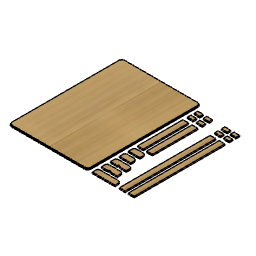
poglos_main_board 211121 (Autodesk Fusion 360 design; units mm, degrees)
Autodesk Fusion 360 part; units mm, degrees
sketch "Main Board" plane through (0, 0, 0) normal (0, 0, 1) x (1, 0, 0)
  line L0 (0, 0) -> (350, 0)
  line L1 (350, 0) -> (350, 500)
  line L2 (350, 500) -> (0, 500)
  line L3 (0, 500) -> (0, 0)
  line L4 (134.9528, 99.915) -> (214.9528, 99.915)
  line L5 (214.9528, 99.915) -> (214.9528, 59.915)
  line L6 (214.9528, 59.915) -> (134.9528, 59.915)
  line L7 (134.9528, 59.915) -> (134.9528, 99.915)
  line L8 (75, 450) -> (275, 450)
  line L9 (275, 450) -> (275, 50)
  line L10 (275, 50) -> (75, 50)
  line L11 (75, 50) -> (75, 450)
  dimension "d1" = 350
  dimension "d2" = 500
  constraint horizontal L0
  constraint vertical L1
  constraint horizontal L2
  constraint vertical L3
  constraint coincident L0.start L3.end
  constraint perpendicular L3 L4
  constraint perpendicular L4 L5
  constraint perpendicular L3 L6
  constraint perpendicular L4 L7
  constraint horizontal L8
  constraint vertical L9
  constraint horizontal L10
  constraint vertical L11
  measures "d1" distance of L0.start L0.end
  measures "d2" distance of L0.start L2.end
extrude "Extrude1" add sketch "Main Board" along normal blind 3 contours L0 L1 L2 L3 | L4 L5 L6 L7 | L8 L9 L10 L11 makes body 1
fillet "Fillet1" radius 15 4 edges at (350, 500, 1.5) (350, 0, 1.5) (0, 0, 1.5) (0, 500, 1.5) on bodies 1
extrude "Extrude2" add 1 faces at (116.6667, 328.3333, 3) along direction (0, 0, 1) blind 3 on bodies 1 bodies 1
chamfer "Chamfer2" distance 2 angle 45 8 edges at (175, 0, 6) (345.6066, 4.3934, 6) (350, 250, 6) (345.6066, 495.6066, 6) (175, 500, 6) (4.3934, 495.6066, 6) (0, 250, 6) (4.3934, 4.3934, 6) on bodies 1
sketch "Support Large" plane through (0, 0, 6) normal (0, 0, 1) x (-1, 0, 0)
  line L0 (-15, -2) -> (-335, -2)
  arc A0 (-335, -2) -> (-348, -15) centre (-335, -15) ccw
  line L1 (-348, -15) -> (-348, -485)
  arc A1 (-348, -485) -> (-335, -498) centre (-335, -485) ccw
  line L2 (-335, -498) -> (-15, -498)
  arc A2 (-15, -498) -> (-2, -485) centre (-15, -485) ccw
  line L3 (-2, -485) -> (-2, -15)
  arc A3 (-2, -15) -> (-15, -2) centre (-15, -15) ccw
  line L4 (-370, 0) -> (-470, 0)
  line L5 (-470, 0) -> (-470, -25)
  line L6 (-470, -25) -> (-370, -25)
  line L7 (-370, -25) -> (-370, 0)
  dimension "d12" = 100
  dimension "d13" = 25
  constraint horizontal L4
  constraint vertical L5
  constraint horizontal L6
  constraint vertical L7
  measures "d12" distance of L4.start L4.end
  measures "d13" distance of L4.start L6.end
sketch "Case Mid" plane through (0, 0, 6) normal (0, 0, 1) x (1, 0, 0)
  line L0 (370, 40) -> (440, 40)
  line L1 (440, 40) -> (440, 65)
  line L2 (440, 65) -> (370, 65)
  line L3 (370, 65) -> (370, 40)
  line L4 (370, 80) -> (440, 80)
  line L5 (440, 80) -> (440, 105)
  line L6 (440, 105) -> (370, 105)
  line L7 (370, 105) -> (370, 80)
  circle A0 centre (405, 80) radius 5
  circle A1 centre (405, 40) radius 5
  dimension "d14" = 70
  dimension "d15" = 25
  dimension "d16" = 70
  dimension "d17" = 25
  dimension "d18" = 10
  dimension "d19" = 10
  constraint horizontal L0
  constraint vertical L1
  constraint horizontal L2
  constraint vertical L3
  constraint horizontal L4
  constraint vertical L5
  constraint horizontal L6
  constraint vertical L7
  constraint midpoint L4 A0.centre
  constraint midpoint L0 A1.centre
  measures "d14" distance of L0.start L0.end
  measures "d15" distance of L0.start L2.end
  measures "d16" distance of L4.start L4.end
  measures "d17" distance of L4.start L6.end
  measures "d18" diameter of A0
  measures "d19" diameter of A1
sketch "Case Small" plane through (0, 0, 0) normal (0, 0, 1) x (1, 0, 0)
  line L0 (370, 120) -> (420, 120)
  line L1 (420, 120) -> (420, 145)
  line L2 (420, 145) -> (370, 145)
  line L3 (370, 145) -> (370, 120)
  line L4 (370, 160) -> (420, 160)
  line L5 (420, 160) -> (420, 185)
  line L6 (420, 185) -> (370, 185)
  line L7 (370, 185) -> (370, 160)
  dimension "d20" = 50
  dimension "d21" = 25
  dimension "d22" = 50
  dimension "d23" = 25
  constraint horizontal L0
  constraint vertical L1
  constraint horizontal L2
  constraint vertical L3
  constraint horizontal L4
  constraint vertical L5
  constraint horizontal L6
  constraint vertical L7
  measures "d20" distance of L0.start L0.end
  measures "d21" distance of L0.start L2.end
  measures "d22" distance of L4.start L4.end
  measures "d23" distance of L4.start L6.end
extrude "Extrude3" add sketch "Support Large" along normal blind 6 separate body contours L4 L5 L6 L7 makes body 2
extrude "Extrude4" add sketch "Case Mid" along normal blind 6 separate body contours L0 L1 L2 L3 A1 | L4 L5 L6 L7 A0 makes body 3 at (405.1246, 58.3287, 6) makes body 4 at (405.1246, 98.3287, 6)
extrude "Extrude5" add sketch "Case Small" along normal blind 6 separate body makes body 5 at (386.6667, 136.6667, 0) makes body 6 at (386.6667, 176.6667, 0)
move_body "Move2" bodies 2 to x (1, 0, 0) y (0, 1, 0) z (0, 0, 1) at (0, 0, -10)
move_body "Move3" bodies 3 4 to x (1, 0, 0) y (0, 1, 0) z (0, 0, 1) at (0, 0, -10)
move_body "Move4" bodies 2 3 4 to x (1, 0, 0) y (0, 1, 0) z (0, 0, 1) at (0, 0, 1)
move_body "Move5" bodies 2 3 4 to x (1, 0, 0) y (0, 1, 0) z (0, 0, 1) at (0, 0, 3)
fillet "Fillet2" radius 10 10 edges at (470, 25, 3) (370, 25, 3) (440, 65, 3) (370, 65, 3) (440, 105, 3) (370, 105, 3) (420, 145, 3) (370, 145, 3) (420, 185, 3) (370, 185, 3) on bodies 2 3 4 5 6
sketch "Wall Long" plane through (0, 0, 6) normal (0, 0, 1) x (-1, 0, 0)
  line L0 (-15, -2) -> (-335, -2)
  arc A0 (-335, -2) -> (-348, -15) centre (-335, -15) ccw
  line L1 (-348, -15) -> (-348, -485)
  arc A1 (-348, -485) -> (-335, -498) centre (-335, -485) ccw
  line L2 (-335, -498) -> (-15, -498)
  arc A2 (-15, -498) -> (-2, -485) centre (-15, -485) ccw
  line L3 (-2, -485) -> (-2, -15)
  arc A3 (-2, -15) -> (-15, -2) centre (-15, -15) ccw
  line L4 (-490, 0) -> (-515, 0)
  line L5 (-515, 0) -> (-515, -400)
  line L6 (-515, -400) -> (-490, -400)
  line L7 (-490, -400) -> (-490, 0)
  dimension "d37" = 25
  dimension "d38" = 400
  constraint horizontal L4
  constraint vertical L5
  constraint horizontal L6
  constraint vertical L7
  measures "d37" distance of L4.start L4.end
  measures "d38" distance of L4.start L6.end
sketch "Wall Short" plane through (0, 0, 0) normal (0, 0, 1) x (1, 0, 0)
  line L0 (370, 200) -> (395, 200)
  line L1 (395, 200) -> (395, 400)
  line L2 (395, 400) -> (370, 400)
  line L3 (370, 400) -> (370, 200)
  dimension "d39" = 25
  dimension "d40" = 200
  constraint horizontal L0
  constraint vertical L1
  constraint horizontal L2
  constraint vertical L3
  measures "d39" distance of L0.start L0.end
  measures "d40" distance of L0.start L2.end
extrude "Extrude8" add sketch "Wall Short" along normal blind 6 separate body makes body 7
extrude "Extrude9" add sketch "Wall Long" along normal blind 6 separate body contours L4 L5 L6 L7 makes body 8
copy_body "CopyPasteBodies2" bodies 7 makes body 9
move_body "Move8" bodies 9 to x (1, 0, 0) y (0, 1, 0) z (0, 0, 1) at (40, 0, 0)
copy_body "CopyPasteBodies3" bodies 8 makes body 10
move_body "Move9" bodies 10 to x (1, 0, 0) y (0, 1, 0) z (0, 0, 1) at (40, 0, 0)
sketch "Sketch9" plane through (0, 0, 0) normal (0, 0, 1) x (1, 0, 0)
  line L0 (370, 420) -> (395, 420)
  line L1 (395, 420) -> (395, 435)
  line L2 (395, 435) -> (370, 435)
  line L3 (370, 435) -> (370, 420)
  dimension "d45" = 25
  dimension "d46" = 15
  constraint horizontal L0
  constraint vertical L1
  constraint horizontal L2
  constraint vertical L3
  measures "d45" distance of L0.start L0.end
  measures "d46" distance of L0.start L2.end
extrude "Extrude10" add sketch "Sketch9" along normal blind 6 separate body makes body 11
copy_body "CopyPasteBodies4" bodies 11 makes body 12
move_body "Move10" bodies 12 to x (1, 0, 0) y (0, 1, 0) z (0, 0, 1) at (0, 30, 0)
copy_body "CopyPasteBodies5" bodies 12 11 makes body 13 makes body 14
move_body "Move11" bodies 13 14 to x (1, 0, 0) y (0, 1, 0) z (0, 0, 1) at (40, 0, 0)
copy_body "CopyPasteBodies6" bodies 11 14 12 13 makes body 15 makes body 16 makes body 17 makes body 18
move_body "Move12" bodies 15 16 17 18 to x (1, 0, 0) y (0, 1, 0) z (0, 0, 1) at (120, 0, 0)
move_body "Move13" bodies 17 15 4 16 14 3 5 8 10 6 12 18 2 1 7 13 11 9 to x (1, 0, 0) y (0, 1, 0) z (0, 0, 1) at (31.3556, 21.3359, 0)
move_body "Move14" bodies 2 16 13 6 1 4 3 17 15 7 11 10 18 14 8 5 12 9 to x (1, 0, 0) y (0, 1, 0) z (0, 0, 1) at (-10.4316, -0.5413, 0)
move_body "Move15" bodies 8 10 to x (1, 0, 0) y (0, 1, 0) z (0, 0, 1) at (0, 0, -6)
extrude "Extrude7" [rolled back] along distance 6 taper angle 0
move_body "Move6" [rolled back]
pasted_body "CopyPasteBodies1" makes body 19
move_body "Move7" [rolled back]
moveface "MoveFace1" [suppressed]
move_body "Move1" [suppressed]
move_face "OffsetFaces1" [suppressed]
named bodies: "Main Board", "Support Large", "Case Mid", "Case Mid 2", "Case Small", "Case Small 2", "Wall Long 1", "Wall Long 2", "Wall Short 1", "Wall Short 2", "Wall Long 1 (1)", "Corner", "Corner (1)", "Corner (2)", "Corner (1) (1)", "Corner (3)", "Corner (2) (1)", "Corner (1) (1) (1)", "Corner (1) (1) (1) (1)"
